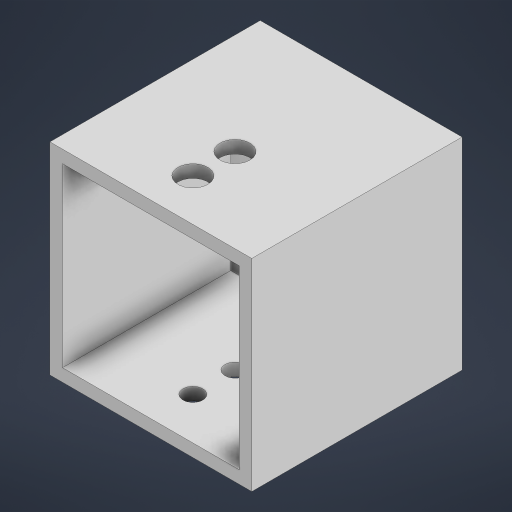
# Autodesk Inventor part: CS_Climb_Inner_Tube_End_Cap
Saved by Autodesk Inventor 2023 (Build 270158000, 158)
## iProperties
Created: 2024-02-19
Part Number: CS_Climb_Inner_Tube_End_Cap
Material: Generic
Document SubType Name: Modeling
Designer: kelle
Density: 1 g/cm^3
Appearance: Default
Author: kelle
Autodesk Inventor part; units mm, degrees
ref_plane "YZ Plane" through (0, 0, 0) normal (1, 0, 0) x (0, 1, 0)
ref_plane "XZ Plane" through (0, 0, 0) normal (0, 1, 0) x (-1, 0, 0)
ref_plane "XY Plane" through (0, 0, 0) normal (0, 0, 1) x (1, 0, 0)
sketch "Sketch1" plane through (0, 0, 0) normal (0, 0, 1) x (1, 0, 0)
  line L0 (13.335, -13.335) -> (-13.335, -13.335)
  line L1 (-13.335, -13.335) -> (-13.335, 13.335)
  line L2 (-13.335, 13.335) -> (13.335, 13.335)
  line L3 (13.335, 13.335) -> (13.335, -13.335)
  line L4 (13.335, -13.335) -> (-13.335, 13.335) construction
  line L5 (-13.335, -13.335) -> (13.335, 13.335) construction
  line L6 (15.24, -15.24) -> (-15.24, -15.24)
  line L7 (-15.24, -15.24) -> (-15.24, 15.24)
  line L8 (-15.24, 15.24) -> (15.24, 15.24)
  line L9 (15.24, 15.24) -> (15.24, -15.24)
  line L10 (15.24, -15.24) -> (-15.24, 15.24) construction
  line L11 (-15.24, -15.24) -> (15.24, 15.24) construction
  point P0 (0, 0)
  dimension "d0" = 26.67
  dimension "d1" = 26.67
  dimension "d2" = 30.48
  dimension "d3" = 30.48
  constraints: 24 end point, 4 midpoint, 4 parallel, 2 horizontal, 2 perpendicular
  measures "d0" distance of L1.end L2.end
  measures "d1" distance of L0.end L1.end
  measures "d2" distance of L7.end L8.end
  measures "d3" distance of L6.end L7.end
extrude "Extrusion1" add sketch "Sketch1" along normal blind 31.75
extrude "Extrusion2" add sketch "Sketch1" along normal blind 6.35 contours L0 L1 L2 L3
sketch "Sketch2" plane through (-15.24, 15.24, 0) normal (0, 1, 0) x (1, 0, 0)
  line L0 (1.905, -6.35) -> (28.575, -6.35) projected
  line L1 (30.48, 0) -> (0, 0) projected
  line L2 (0, 0) -> (0, -31.75) projected
  line L3 (30.48, -31.75) -> (0, -31.75) projected
  line L4 (30.48, 0) -> (30.48, -31.75) projected
  line L5 (15.24, 0) -> (15.24, -31.75) construction
  line L6 (28.575, -31.75) -> (1.905, -31.75) construction
  circle A0 centre (15.24, -19.05) radius 2.25
  circle A1 centre (15.24, -25.4) radius 2.25
  dimension "d8" = 4.5
  dimension "d9" = 12.7
  dimension "d10" = 4.5
  dimension "d11" = 6.35
  constraints: 2 centre point, 2 end point, 2 point on line, 1 midpoint
  measures "d8" diameter of A0
  measures "d9" distance from line of L0 A0.centre
  measures "d10" diameter of A1
  measures "d11" distance of A0.centre A1.centre
extrude "Extrusion3" cut sketch "Sketch2" against normal up to surface (28.575 mm away) contours A0 | A1
sketch "Sketch3" plane through (-15.24, -15.24, 0) normal (0, -1, 0) x (1, 0, 0)
  circle A0 centre (15.24, 19.05) radius 2.25 projected
  line L0 (0, 0) -> (30.48, 0) projected
  line L1 (30.48, 0) -> (30.48, 31.75) projected
  line L2 (0, 31.75) -> (30.48, 31.75) projected
  line L3 (0, 0) -> (0, 31.75) projected
  circle A1 centre (15.24, 25.4) radius 2.25 projected
  circle A2 centre (15.24, 25.4) radius 1.5
  circle A3 centre (15.24, 19.05) radius 1.5
  point P0 (15.24, 0)
  dimension "d14" = 3
  dimension "d15" = 3
  constraints: 2 centre point, 2 coincident
  measures "d14" diameter of A2
  measures "d15" diameter of A3
extrude "Extrusion4" cut sketch "Sketch3" against normal up to surface (28.575 mm away) contours A2 | A3
body "Solid1"
